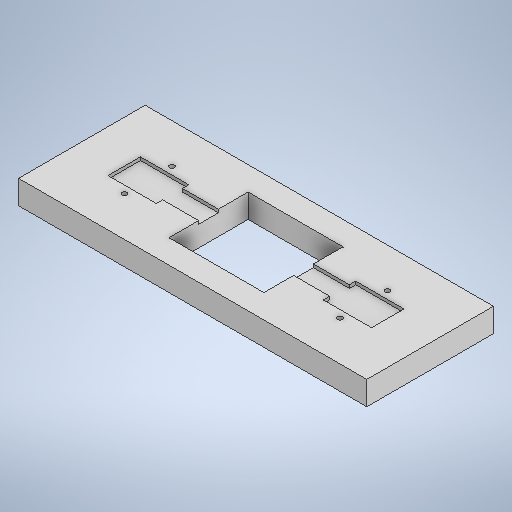
# Autodesk Inventor part: Grundplatte_v2
Saved by Autodesk Inventor 2025 (Build 290162000, 162)
## iProperties
Created: 2026-06-23
Part Number: Grundplatte_v2
Material: Generisch
Document SubType Name: Modeling
Designer: GemmiDad-GBSE
Density: 1 g/cm^3
Appearance: Vorgabe
Author: GemmiDad-GBSE
Autodesk Inventor part; units mm, degrees
ref_plane "YZ Plane" through (0, 0, 0) normal (1, 0, 0) x (0, 1, 0)
ref_plane "XZ Plane" through (0, 0, 0) normal (0, 1, 0) x (-1, 0, 0)
sketch "Skizze1" plane through (0, 0, 0) normal (0, 0, 1) x (1, 0, 0)
  line L0 (-110, -40) -> (110, -40)
  line L1 (110, -40) -> (110, 40)
  line L2 (110, 40) -> (-110, 40)
  line L3 (-110, 40) -> (-110, -40)
  constraints: 8 end point, 2 parallel, 1 horizontal, 1 perpendicular
extrude "Extrusion1" add sketch "Skizze1" along normal blind 15
ref_plane "Arbeitsebene1" through (0, 0, 15) normal (0, 0, 1) x (1, 0, 0)
sketch "Skizze2" plane through (0, 0, 15) normal (0, 0, 1) x (1, 0, 0)
  line L0 (-83.25, -10.25) -> (-52.75, -10.25)
  line L1 (-52.75, -10.25) -> (-52.75, 10.25)
  line L2 (-52.75, 10.25) -> (-83.25, 10.25)
  line L3 (-83.25, 10.25) -> (-83.25, -10.25)
  constraints: 8 end point, 2 parallel, 1 horizontal, 1 perpendicular
extrude "Extrusion2" cut sketch "Skizze2" against normal blind 2
sketch "Skizze3" plane through (0, 0, 15) normal (0, 0, 1) x (1, 0, 0)
  line L0 (52.75, -10.25) -> (83.25, -10.25)
  line L1 (83.25, -10.25) -> (83.25, 10.25)
  line L2 (83.25, 10.25) -> (52.75, 10.25)
  line L3 (52.75, 10.25) -> (52.75, -10.25)
  constraints: 8 end point, 2 parallel, 1 horizontal, 1 perpendicular
extrude "Extrusion3" cut sketch "Skizze3" against normal blind 2
sketch "Skizze4" plane through (0, 0, 15) normal (0, 0, 1) x (1, 0, 0)
  line L0 (-53.25, -6.25) -> (53.25, -6.25)
  line L1 (53.25, -6.25) -> (53.25, 6.25)
  line L2 (53.25, 6.25) -> (-53.25, 6.25)
  line L3 (-53.25, 6.25) -> (-53.25, -6.25)
  constraints: 8 end point, 2 parallel, 1 horizontal, 1 perpendicular
extrude "Extrusion4" cut sketch "Skizze4" against normal blind 2
sketch "Skizze5" plane through (0, 0, 15) normal (0, 0, 1) x (1, 0, 0)
  line L0 (-30, -25) -> (30, -25)
  line L1 (30, -25) -> (30, 25)
  line L2 (30, 25) -> (-30, 25)
  line L3 (-30, 25) -> (-30, -25)
  constraints: 8 end point, 2 parallel, 1 horizontal, 1 perpendicular
extrude "Extrusion5" cut sketch "Skizze5" against normal blind 16
sketch "Skizze6" plane through (0, 0, 15) normal (0, 0, 1) x (1, 0, 0)
  circle A0 centre (-68, -15) radius 1.6
  circle A1 centre (-68, 15) radius 1.6
  circle A2 centre (68, -15) radius 1.6
  circle A3 centre (68, 15) radius 1.6
  constraints: 4 centre point
extrude "Extrusion6" cut sketch "Skizze6" against normal blind 16
